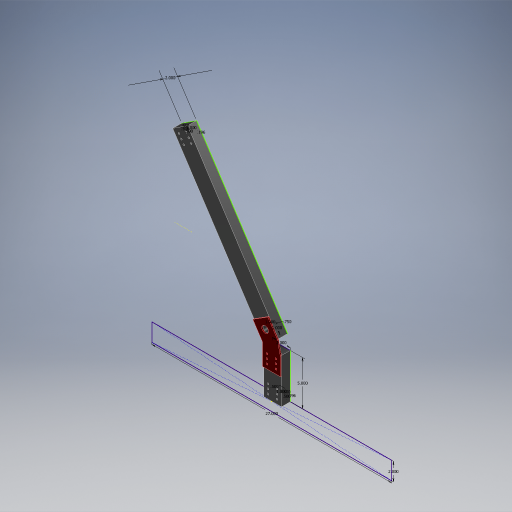
# Autodesk Inventor part: temp
Saved by Autodesk Inventor 2024.2 (Build 282272000, 272)
## iProperties
Created: 2024-01-20
Part Number: temp
Material: Aluminum 6061
Document SubType Name: Modeling
Designer: rohan
Density: 2.7 g/cm^3
Appearance: Aluminum - Flat
Author: rohan
Autodesk Inventor part; units mm, degrees
ref_plane "YZ Plane" through (0, 0, 0) normal (1, 0, 0) x (0, 1, 0)
ref_plane "XZ Plane" through (0, 0, 0) normal (0, 1, 0) x (-1, 0, 0)
ref_plane "XY Plane" through (0, 0, 0) normal (0, 0, 1) x (1, 0, 0)
sketch "Sketch1" plane through (0, 0, 0) normal (0, 0, 1) x (1, 0, 0)
  line L0 (-342.9, 25.4) -> (342.9, 25.4)
  line L1 (342.9, 25.4) -> (342.9, -25.4)
  line L2 (342.9, -25.4) -> (-342.9, -25.4)
  line L3 (-342.9, -25.4) -> (-342.9, 25.4)
  line L4 (-342.9, 25.4) -> (342.9, -25.4) construction
  line L5 (342.9, 25.4) -> (-342.9, -25.4) construction
  line L6 (-277.1742, 25.4) -> (-226.3742, 25.4)
  line L7 (2.2258, 25.4) -> (53.0258, 25.4)
  line L8 (53.0258, 25.4) -> (53.0258, 152.4)
  line L9 (53.0258, 152.4) -> (2.2258, 152.4)
  line L10 (2.2258, 152.4) -> (2.2258, 25.4)
  circle A0 centre (14.9258, 38.1) radius 2.4892
  circle A1 centre (40.3258, 38.1) radius 2.4892
  circle A2 centre (14.9258, 50.8) radius 2.4892
  circle A3 centre (40.3258, 50.8) radius 2.4892
  circle A4 centre (14.9258, 63.5) radius 2.4892
  circle A5 centre (40.3258, 63.5) radius 2.4892
  line L11 (-277.1742, 304.8) -> (-226.3742, 304.8) construction
  line L12 (-257.897, 559.7678) -> (-215.379, 587.5681)
  line L13 (-215.379, 587.5681) -> (44.749, 189.7254)
  line L14 (44.749, 189.7254) -> (2.2309, 161.9251)
  line L15 (2.2309, 161.9251) -> (-257.897, 559.7678)
  circle A6 centre (-240.3174, 556.0884) radius 2.4892
  circle A7 centre (-219.0584, 569.9885) radius 2.4892
  circle A8 centre (-233.3674, 545.4589) radius 2.4892
  circle A9 centre (-212.1084, 559.359) radius 2.4892
  circle A10 centre (-226.4173, 534.8293) radius 2.4892
  circle A11 centre (-205.1583, 548.7295) radius 2.4892
  circle A12 centre (9.5898, 197.0843) radius 9.525
  line L16 (2.2258, 88.9) -> (53.0258, 88.9) construction
  circle A13 centre (14.9258, 139.7) radius 2.4892
  circle A14 centre (40.3258, 139.7) radius 2.4892
  circle A15 centre (14.9258, 127) radius 2.4892
  circle A16 centre (40.3258, 127) radius 2.4892
  circle A17 centre (14.9258, 114.3) radius 2.4892
  circle A18 centre (40.3258, 114.3) radius 2.4892
  point P0 (0, 0)
  point P1 (53.0258, 25.4)
  dimension "d0" = 685.8
  dimension "d1" = 50.8
  dimension "d5" = 127
  dimension "d21" = 4.9784
  dimension "d22" = 12.7
  dimension "d23" = 12.7
  dimension "d26" = 25.4
  dimension "d29" = 12.7
  dimension "d60" = 50.8
  dimension "d61" = 50.8
  dimension "d62" = 4.9784
  dimension "d63" = 12.7
  dimension "d64" = 12.7
  dimension "d67" = 25.4
  dimension "d70" = 12.7
  dimension "d73" = 19.05
  dimension "d74" = 25.4
  dimension "d75" = 25.4
  constraints: 34 end point, 19 centre point, 6 parallel, 6 symmetric about line, 4 horizontal, 4 midpoint, 3 perpendicular, 2 point on line, 1 vertical, 28 other
  measures "d0" distance of L1.end L2.end
  measures "d1" distance of L0.end L1.end
  measures "d5" distance of L8.end L7.end
  measures "d21" diameter of A0
  measures "d22" distance from line of L10 A0.centre
  measures "d23" distance from line of A0.centre L0
  measures "d26" distance of A0.centre A1.centre
  measures "d29" distance of A0.centre A2.centre
  measures "d60" distance of L12.start L12.end
  measures "d61" distance of L8.end L9.end
  measures "d62" diameter of A6
  measures "d63" distance from line of A6.centre L12
  measures "d64" distance from line of L15 A6.centre
  measures "d67" distance of A6.centre A7.centre
  measures "d70" distance of A6.centre A8.centre
  measures "d73" diameter of A12
  measures "d74" distance from line of A12.centre L15
  measures "d75" distance from line of A12.centre L14
extrude "Extrusion8" add sketch "Sketch1" along normal blind 25.4 contours L12 L13 L14 L15
extrude "Extrusion9" add sketch "Sketch1" along normal blind 25.4 separate body contours L10 L9 L8 L0
sketch "Sketch7" plane through (0, 0, 25.4) normal (0, 0, 1) x (1, 0, 0)
  line L0 (2.2309, 161.9251) -> (44.749, 189.7254) projected
  line L1 (44.749, 189.7254) -> (-215.379, 587.5681) projected
  line L2 (-215.379, 587.5681) -> (-257.897, 559.7678) projected
  line L3 (-257.897, 559.7678) -> (2.2309, 161.9251) projected
  circle A0 centre (9.5898, 197.0843) radius 9.525 projected
  circle A1 centre (-205.1583, 548.7295) radius 2.4892 projected
  circle A2 centre (-226.4173, 534.8293) radius 2.4892 projected
  circle A3 centre (-212.1084, 559.359) radius 2.4892 projected
  circle A4 centre (-233.3674, 545.4589) radius 2.4892 projected
  circle A5 centre (-219.0584, 569.9885) radius 2.4892 projected
  circle A6 centre (-240.3174, 556.0884) radius 2.4892 projected
  line L4 (2.2258, 152.4) -> (2.2258, 25.4) projected
  line L5 (2.2258, 25.4) -> (53.0258, 25.4) projected
  line L6 (53.0258, 25.4) -> (53.0258, 152.4) projected
  line L7 (53.0258, 152.4) -> (2.2258, 152.4) projected
  circle A7 centre (40.3258, 139.7) radius 2.4892 projected
  circle A8 centre (40.3258, 114.3) radius 2.4892 projected
  circle A9 centre (14.9258, 127) radius 2.4892 projected
  circle A10 centre (14.9258, 38.1) radius 2.4892 projected
  circle A11 centre (40.3258, 38.1) radius 2.4892 projected
  circle A12 centre (14.9258, 50.8) radius 2.4892 projected
  circle A13 centre (40.3258, 50.8) radius 2.4892 projected
  circle A14 centre (14.9258, 63.5) radius 2.4892 projected
  circle A15 centre (40.3258, 63.5) radius 2.4892 projected
  circle A16 centre (40.3258, 127) radius 2.4892 projected
  circle A17 centre (14.9258, 114.3) radius 2.4892 projected
  circle A18 centre (14.9258, 139.7) radius 2.4892 projected
  line L8 (2.2258, 152.4) -> (2.2309, 161.9251)
  line L9 (2.2309, 161.9251) -> (-25.5694, 204.4432)
  line L10 (-257.897, 559.7678) -> (2.2309, 161.9251) projected
  line L11 (-25.5694, 204.4432) -> (17.415, 231.5303)
  line L12 (17.415, 231.5303) -> (44.749, 189.7254)
  line L13 (44.749, 189.7254) -> (53.0258, 152.4)
  line L14 (53.0258, 152.4) -> (53.0258, 101.6)
  line L15 (53.0258, 25.4) -> (53.0258, 152.4) projected
  line L16 (53.0258, 101.6) -> (2.2258, 101.6)
  line L17 (2.2258, 152.4) -> (2.2258, 25.4) projected
  line L18 (2.2258, 101.6) -> (2.2258, 152.4)
  point P0 (0, 0)
  dimension "d80" = 50.8
  dimension "d81" = 50.8
  constraints: 16 end point, 4 point on line, 2 perpendicular, 1 collinear
  measures "d80" distance of L0.start L9.end
  measures "d81" distance of L6.end L14.end
extrude "Extrusion10" add sketch "Sketch7" along normal blind 3.175 separate body contours L3 L11 L1 L0 | L0 L13 L7 L8 | L7 L6 L16 L4
body "Solid4"
body "Solid5"
body "Solid6"
